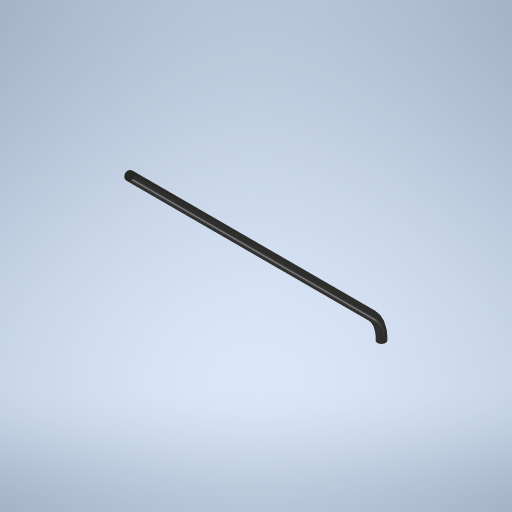
# Autodesk Inventor part: cable 45°
Saved by Autodesk Inventor 2023 (Build 270158000, 158)
## iProperties
Created: 2022-10-27
Part Number: cable 45°
Material: Generic
Document SubType Name: Modeling
Designer: Xiaba
Density: 1 g/cm^3
Appearance: Default
Author: Xiaba
Autodesk Inventor part; units mm, degrees
ref_plane "YZ Plane" through (0, 0, 0) normal (1, 0, 0) x (0, 1, 0)
ref_plane "XZ Plane" through (0, 0, 0) normal (0, 1, 0) x (-1, 0, 0)
ref_plane "XY Plane" through (0, 0, 0) normal (0, 0, 1) x (1, 0, 0)
sketch "Sketch1" plane through (0, 0, 0) normal (0, 1, 0) x (-1, 0, 0)
  circle A0 centre (0, 0) radius 0.25
  dimension "d0" = 0.5
  constraints: 1 centre point, 1 coincident
  measures "d0" diameter of A0
sketch "Sketch2" plane through (0, 0, 0) normal (1, 0, 0) x (0, 1, 0)
  line L0 (0, 0) -> (0.1716, 0)
  line L1 (1.5858, 0.5858) -> (16, 15)
  arc A0 (0.1716, 0) -> (1.5858, 0.5858) centre (0.1716, 2) ccw
  point P0 (1, 0)
  dimension "d1" = 1
  dimension "d2" = 135
  dimension "d3" = 15
  dimension "d9" = 2
  constraints: 4 end point, 2 point on circle, 2 point on line, 2 tangent, 1 centre point, 1 horizontal
  measures "d1" distance of L0.start point (1, 0)
  measures "d2" angle of L0 L1
  measures "d3" horizontal distance of point (1, 0) L1.end
  measures "d9" radius of A0
sweep "Sweep3" add profiles "Sketch1" path "Sketch2"
body "Solid3"
